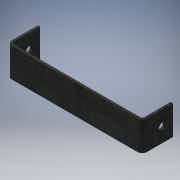
# Autodesk Inventor part: cup
Saved by Autodesk Inventor 2018 (Build 220112000, 112)
## iProperties
Created: 2018-04-05
Part Number: cup
Material: アルミニウム 6061
Document SubType Name: Sheet Metal
Designer: NaMACHAN
Density: 2.7 g/cm^3
Sheet Metal Rule: Default_mm
Appearance: アルミニウム - フラット
Author: NaMACHAN
Autodesk Inventor part; units mm, degrees
ref_plane "YZ Plane" through (0, 0, 0) normal (1, 0, 0) x (0, 1, 0)
ref_plane "XZ Plane" through (0, 0, 0) normal (0, 1, 0) x (-1, 0, 0)
ref_plane "XY Plane" through (0, 0, 0) normal (0, 0, 1) x (1, 0, 0)
sketch "スケッチ1" plane through (0, 0, 0) normal (0, 1, 0) x (-1, 0, 0)
  line L0 (-44, -9.5) -> (44, -9.5)
  line L1 (44, -9.5) -> (44, 9.5)
  line L2 (44, 9.5) -> (-44, 9.5)
  line L3 (-44, 9.5) -> (-44, -9.5)
  line L4 (-44, -9.5) -> (44, 9.5) construction
  line L5 (44, -9.5) -> (-44, 9.5) construction
  point P0 (0, 0)
  dimension "d0" = 88
  dimension "d1" = 19
  measures "d0" distance of L2.end L1.end
  measures "d1" distance of L0.end L1.end
extrude "プレート1" add sketch "スケッチ1" along normal blind 1.5
sketch "スケッチ2" plane through (42.5, 0, -9.5) normal (1, 0, 0) x (0, 1, 0)
  line L0 (0, 19) -> (0, 0)
  line L1 (0, 0) -> (20, 0)
  line L2 (20, 0) -> (20, 19)
  line L3 (20, 19) -> (0, 19)
  constraints: 6 end point, 1 horizontal, 1 perpendicular, 1 vertical
edge flange "フランジ1" height 20 angle 90 thickness 1.5 bend radius 1.5 thickness toward (1, 0, 0) relief straight relief width 1.5 relief depth 0.75 edges at (44, 1.5, 0) wall of the first edge with corners at (42.5, 0, 9.5) (42.5, 0, -9.5) (42.5, 20, -9.5) (42.5, 20, 9.5)
bend "曲げ1"
corner "コーナー1"
sketch "スケッチ3" plane through (-42.5, 0, 9.5) normal (-1, 0, 0) x (0, -1, 0)
  line L0 (0, -19) -> (0, 0)
  line L1 (0, 0) -> (-20, 0)
  line L2 (-20, 0) -> (-20, -19)
  line L3 (-20, -19) -> (0, -19)
  constraints: 6 end point, 1 horizontal, 1 perpendicular, 1 vertical
edge flange "フランジ2" height 20 angle 90 thickness 1.5 bend radius 1.5 thickness toward (-1, 0, 0) relief straight relief width 1.5 relief depth 0.75 edges at (-44, 1.5, 0) wall of the first edge with corners at (-42.5, 0, -9.5) (-42.5, 0, 9.5) (-42.5, 20, 9.5) (-42.5, 20, -9.5)
bend "曲げ2"
corner "コーナー2"
sketch "スケッチ5" plane through (0, 0, 0) normal (0, -1, 0) x (1, 0, 0)
  arc A0 (-35, 2) -> (-35, -2) centre (-35, 0) ccw
  arc A1 (35, -2) -> (35, 2) centre (35, 0) ccw
  line L0 (-35, 2) -> (35, 2)
  line L1 (35, -2) -> (-35, -2)
  point P0 (0, 0)
  dimension "d31" = 4
  dimension "d32" = 2
  dimension "d33" = 2
  dimension "d34" = 2
  dimension "d35" = 35
  dimension "d36" = 35
  constraints: 4 end point, 4 point on circle, 2 centre point, 2 horizontal, 2 vertical alignment
  measures "d31" distance between parallel lines of L0 L1
  measures "d32" radius of A1
  measures "d33" radius of A0
  measures "d34" distance from line of L0 point (0, 0)
  measures "d35" distance of point (0, 0) A0.centre
  measures "d36" distance of A1.centre point (0, 0)
extrude "押し出し1" cut sketch "スケッチ5" against normal blind 1.5
sketch "スケッチ6" plane through (44, 20, 9.5) normal (1, 0, 0) x (0, 0, -1)
  point P0 (9.5, -20)
sketch "スケッチ7" plane through (44, 20, 9.5) normal (1, 0, 0) x (0, 0, -1)
  line L0 (4, -2) -> (15, -2)
  arc A0 (15, -6) -> (15, -2) centre (15, -4) ccw
  line L1 (15, -6) -> (4, -6)
  arc A1 (4, -2) -> (4, -6) centre (4, -4) ccw
  line L2 (0, 0) -> (19, 0) projected
  line L3 (0, -17) -> (0, 0) projected
  line L4 (19, 0) -> (19, -17) projected
  point P0 (9.5, -20)
  dimension "d39" = 2
  dimension "d40" = 4
  dimension "d41" = 4
  dimension "d42" = 4
  constraints: 4 end point, 4 point on circle, 4 tangent, 2 centre point, 1 horizontal, 1 parallel
  measures "d39" radius of A1
  measures "d40" distance from line of L2 A1.centre
  measures "d41" distance from line of L3 A1.centre
  measures "d42" distance from line of L4 A0.centre
extrude "押し出し2" cut sketch "スケッチ7" against normal blind 100
equation "\"d2\" = Thickness"
equation "\"d3\" = BendReliefWidth"
equation "\"d4\" = BendReliefDepth"
equation "\"d5\" = MinimumRemnant"
equation "\"d6\" = TransitionRadius"
equation "\"d9\" = BendRadius"
equation "\"d10\" = CornerReliefSize"
equation "\"d11\" = GapSize"
equation "\"d12\" = JacobiRadiusSize"
equation "\"d13\" = BendReliefWidth"
equation "\"d14\" = BendReliefDepth"
equation "\"d15\" = MinimumRemnant"
equation "\"d16\" = TransitionRadius"
equation "\"d19\" = BendRadius"
equation "\"d20\" = CornerReliefSize"
equation "\"d21\" = GapSize"
equation "\"d22\" = JacobiRadiusSize"
equation "\"BendRadius\" = Thickness"
equation "\"BendReliefWidth\" = Thickness"
equation "\"BendReliefDepth\" = 0.5 * Thickness"
equation "\"CornerReliefSize\" = 4 * Thickness"
equation "\"MinimumRemnant\" = 2 * Thickness"
equation "\"TransitionRadius\" = BendRadius"
equation "\"JacobiRadiusSize\" = BendRadius"
equation "\"GapSize\" = Thickness"
equation "\"Thickness\" = 1.5"
